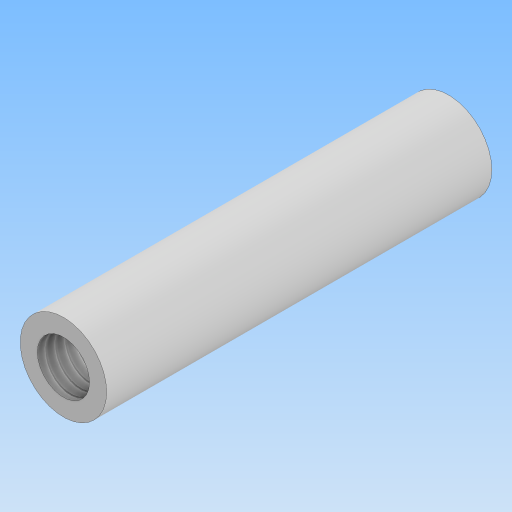
# Autodesk Inventor part: RadBolzen
Saved by Autodesk Inventor 2024.4 (Build 284460000, 460)
## iProperties
Created: 2026-01-05
Part Number: RadBolzen
Material: Generisch
Document SubType Name: Modeling
Designer: windows-desktop
Density: 1 g/cm^3
Appearance: Vorgabe
Mass: 3.6388 g
Surface Area: 24.7965 cm^2
Volume: 3.6388 cm^3
Masse[kg]: 0,004 kg
Author: windows-desktop
Autodesk Inventor part; units mm, degrees
ref_plane "YZ Plane" through (0, 0, 0) normal (1, 0, 0) x (0, 1, 0)
ref_plane "XZ Plane" through (0, 0, 0) normal (0, 1, 0) x (-1, 0, 0)
ref_plane "XY Plane" through (0, 0, 0) normal (0, 0, 1) x (1, 0, 0)
sketch "Skizze1" plane through (0, 0, 0) normal (0, 0, 1) x (1, 0, 0)
  circle A0 centre (0, 0) radius 5.5
  dimension "d0" = 11
  constraints: 1 centre point, 1 coincident
  measures "d0" diameter of A0
extrude "Extrusion1" add sketch "Skizze1" along normal mid plane 49
sketch "Skizze2" plane through (0, 0, 24.5) normal (0, 0, 1) x (1, 0, 0)
  circle A0 centre (0, 0) radius 5.5 construction
  constraints: 1 coincident
hole "Bohrung1" at (0, 0, 24.5) direction (0, 0, -1) diameter 6.647 depth 14 tip angle 118 thread size "M8x1.25" class "6H" standard "ISO Metric profile"
sketch "Skizze3" plane through (0, 0, -24.5) normal (0, 0, -1) x (-1, 0, 0)
  circle A0 centre (0, 0) radius 5.5 construction
  constraints: 1 coincident
hole "Bohrung2" at (0, 0, -24.5) direction (0, 0, 1) diameter 6.647 depth 14 tip angle 118 thread size "M8x1.25" class "6H" standard "ISO Metric profile"
